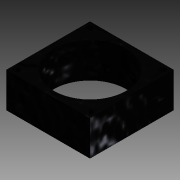
# Autodesk Inventor part: Fan60
Saved by Autodesk Inventor 2014 (Build 180170000, 170)
## iProperties
Created: 2015-04-18
Part Number: Fan60
Material: Generic
Document SubType Name: Modeling
Designer: Owner
Density: 1 g/cm^3
Appearance: Black
Author: Owner
Autodesk Inventor part; units mm, degrees
ref_plane "YZ Plane" through (0, 0, 0) normal (1, 0, 0) x (0, 1, 0)
ref_plane "XZ Plane" through (0, 0, 0) normal (0, 1, 0) x (-1, 0, 0)
ref_plane "XY Plane" through (0, 0, 0) normal (0, 0, 1) x (1, 0, 0)
sketch "Sketch1" plane through (0, 0, 0) normal (0, 1, 0) x (-1, 0, 0)
  line L0 (17.6552, 44.8276) -> (77.6552, 44.8276)
  line L1 (77.6552, 44.8276) -> (77.6552, -15.1724)
  line L2 (77.6552, -15.1724) -> (17.6552, -15.1724)
  line L3 (17.6552, -15.1724) -> (17.6552, 44.8276)
  point P0 (0, 0)
  dimension "d0" = 60
  dimension "d1" = 60
  constraints: 8 end point, 2 parallel, 1 horizontal, 1 perpendicular
  measures "d0" distance of L0.start L0.end
  measures "d1" distance of L0.end L1.end
extrude "Extrusion1" add sketch "Sketch1" along normal blind 25
sketch "Sketch2" plane through (0, 25, 0) normal (0, 1, 0) x (1, 0, 0)
  line L0 (-17.6552, -44.8276) -> (-17.6552, 15.1724) projected
  line L1 (-17.6552, 15.1724) -> (-77.6552, 15.1724) projected
  line L2 (-77.6552, 15.1724) -> (-77.6552, -44.8276) projected
  circle A0 centre (-47.6552, -14.8276) radius 26
  circle A1 centre (-73.6552, 11.1724) radius 2.15
  circle A2 centre (-21.6552, 11.1724) radius 2.15
  circle A3 centre (-21.6552, -40.8276) radius 2.15
  circle A4 centre (-73.6552, -40.8276) radius 2.15
  point P0 (0, 0)
  dimension "d4" = 52
  dimension "d5" = 30
  dimension "d6" = 30
  dimension "d7" = 4.3
  dimension "d8" = 4.3
  dimension "d9" = 4.3
  dimension "d10" = 4.3
  dimension "d11" = 52
  dimension "d12" = 52
  dimension "d13" = 52
  dimension "d14" = 52
  dimension "d15" = 4
  dimension "d16" = 4
  dimension "d17" = 4
  dimension "d18" = 4
  constraints: 5 centre point
  measures "d4" diameter of A0
  measures "d5" distance from line of L0 A0.centre
  measures "d6" distance from line of L1 A0.centre
  measures "d7" diameter of A3
  measures "d8" diameter of A4
  measures "d9" diameter of A1
  measures "d10" diameter of A2
  measures "d11" distance of A2.centre A3.centre
  measures "d12" distance of A4.centre A1.centre
  measures "d13" distance of A3.centre A4.centre
  measures "d14" distance of A2.centre A1.centre
  measures "d15" distance from line of L1 A2.centre
  measures "d16" distance from line of L2 A1.centre
  measures "d17" distance from line of L1 A1.centre
  measures "d18" distance from line of L0 A3.centre
extrude "Extrusion2" cut sketch "Sketch2" against normal blind 38
body "Solid1"
